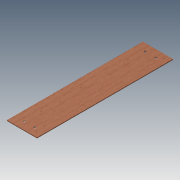
# Autodesk Inventor part: gabarito-bloco-solenoide
Saved by Autodesk Inventor 2017 (Build 210142000, 142)
## iProperties
Created: 2018-08-29
Part Number: gabarito-bloco-solenoide
Material: Wood (Oak)
Document SubType Name: Sheet Metal
Designer: Luiz Gustavo
Density: 0.76 g/cm^3
Sheet Metal Rule: Default_mm
Appearance: White Oak - Natural Medium Gloss
Author: Luiz Gustavo
Autodesk Inventor part; units mm, degrees
ref_plane "YZ Plane" through (0, 0, 0) normal (1, 0, 0) x (0, 1, 0)
ref_plane "XZ Plane" through (0, 0, 0) normal (0, 1, 0) x (-1, 0, 0)
ref_plane "XY Plane" through (0, 0, 0) normal (0, 0, 1) x (1, 0, 0)
sketch "Sketch1" plane through (0, 0, 0) normal (0, 0, 1) x (1, 0, 0)
  circle A0 centre (0.0625, 529.5) radius 2.25
  circle A1 centre (21.0625, 529.5) radius 2.25
  circle A2 centre (0.0625, 770.5) radius 2.25
  circle A3 centre (21.0625, 770.5) radius 2.25
  line L0 (40.5624, -111.2599) -> (40.5624, 1344.9999)
  line L1 (-19.4375, -111.2599) -> (-19.4375, 1344.9999)
  line L2 (-19.4375, 785.5) -> (40.5624, 785.5)
  line L3 (40.5624, 785.5) -> (40.5624, 514.5)
  line L4 (40.5624, 514.5) -> (-19.4375, 514.5)
  line L5 (-19.4375, 514.5) -> (-19.4375, 785.5)
  circle A4 centre (21.0625, 770.5) radius 2.25
  circle A5 centre (0.0625, 770.5) radius 2.25
  circle A6 centre (21.0625, 529.5) radius 2.25
  circle A7 centre (0.0625, 529.5) radius 2.25
  point P0 (0, 0)
  dimension "d0" = 15
  dimension "d1" = 15
  measures "d0" distance from line of L4 A1.centre
  measures "d1" distance from line of A3.centre L2
extrude "Plate1" add sketch "Sketch1" along normal blind 1.5
equation "\"d1\" = d0"
equation "\"BendRadius\" = Thickness"
equation "\"BendReliefWidth\" = Thickness"
equation "\"BendReliefDepth\" = 0.5 * Thickness"
equation "\"CornerReliefSize\" = 4 * Thickness"
equation "\"MinimumRemnant\" = 2 * Thickness"
equation "\"TransitionRadius\" = BendRadius"
equation "\"JacobiRadiusSize\" = BendRadius"
equation "\"GapSize\" = Thickness"
equation "\"d2\" = BendRadius"
equation "\"Thickness\" = 1.5"
body "Solid1"
